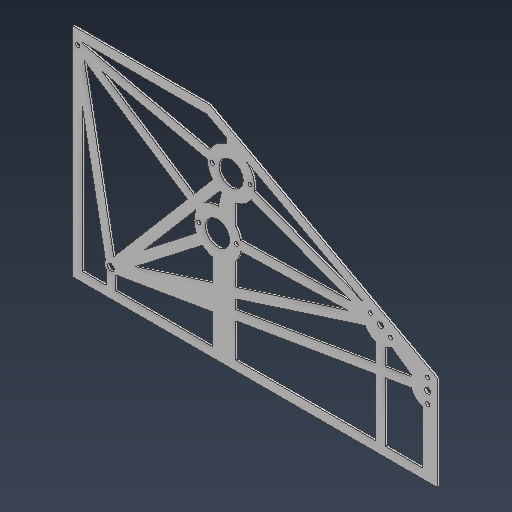
# Autodesk Inventor part: стенка
Saved by Autodesk Inventor 2025 (Build 290162000, 162)
## iProperties
Created: 2025-10-03
Part Number: стенка
Material: Типовые
Document SubType Name: Modeling
Designer: Phantom
Density: 1 g/cm^3
Appearance: По умолчанию
Author: Phantom
Autodesk Inventor part; units mm, degrees
ref_plane "YZ Plane" through (0, 0, 0) normal (1, 0, 0) x (0, 1, 0)
ref_plane "XZ Plane" through (0, 0, 0) normal (0, 1, 0) x (-1, 0, 0)
ref_plane "XY Plane" through (0, 0, 0) normal (0, 0, 1) x (1, 0, 0)
sketch "Эскиз1" plane through (0, 0, 0) normal (0, 0, 1) x (1, 0, 0)
  line L0 (0, 0) -> (380, 0)
  line L1 (380, 0) -> (380, 227)
  line L2 (380, 227) -> (0, 227)
  line L3 (0, 227) -> (0, 0)
  dimension "d0" = 380
  dimension "d1" = 227
  constraints: 8 end point, 2 parallel, 1 horizontal, 1 perpendicular
  measures "d0" distance of L2.end L1.end
  measures "d1" distance of L1.end L0.end
extrude "Выдавливание1" add sketch "Эскиз1" along normal blind 2
sketch "Эскиз2" plane through (0, 0, 2) normal (0, 0, 1) x (1, 0, 0)
  arc A0 (28.7106, 220.3235) -> (184.1593, 0) centre (184.1593, 165) ccw projected
  line L0 (380, 0) -> (380, 227) projected
  line L1 (380, 227) -> (0, 227) projected
  line L2 (0, 227) -> (0, 0) projected
  line L3 (0, 0) -> (380, 0) projected
  line L4 (19.1593, 227.9564) -> (19.1593, -26.9054)
  line L5 (0, 227) -> (0, 0) projected
  circle A1 centre (184.1593, 165) radius 165
  point P0 (19.1593, 165)
  point P1 (24, 227)
  point P2 (19.1593, 0)
  point P3 (19.1593, 227)
  point P4 (184.1593, 0)
  point P5 (28.7106, 220.3235)
  point P6 (31.2508, 227)
  constraints: 2 end point, 1 centre point, 1 coincident, 1 concentric, 1 parallel, 1 tangent
extrude "Выдавливание2" cut sketch "Эскиз2" against normal blind 10 contours L4 L3 L2 L1
sketch "Эскиз3" plane through (0, 0, 0) normal (0, 0, -1) x (-1, 0, 0)
  line L0 (-232.105, -3.3128) -> (-396.3335, -92) projected
  line L1 (-142.3437, 227) -> (-503.0133, 32.2299)
  line L2 (-14.2955, 176.8048) -> (-380, 176.8048) projected
  line L3 (-14.2955, 180) -> (-380, 180) projected
  line L4 (-380, 0) -> (-380, 176.8048) projected
  line L5 (-14.1593, 0) -> (-380, 0) projected
  line L6 (-14.1593, 0) -> (-14.1593, 170) projected
  arc A0 (-14.1593, 170) -> (-14.2955, 176.8048) centre (-184.1593, 170) ccw projected
  line L7 (-19.1593, 0) -> (-19.1593, 227) projected
  line L8 (-380, 227) -> (-19.1593, 227) projected
  line L9 (-380, 0) -> (-380, 227) projected
  line L10 (-19.1593, 0) -> (-380, 0) projected
  point P0 (0, 0)
  point P1 (-380, 98.66)
  dimension "d6" = 160
  constraints: 2 end point, 1 horizontal alignment, 1 parallel, 1 point on line, 1 other
  measures "d6" distance between parallel lines of L0 L1
extrude "Выдавливание3" cut sketch "Эскиз3" against normal blind 10 contours L1 L3 L9 L8 | L1 L2 L9 L3 | L1 L4 L2
sketch "Эскиз4" plane through (0, 0, 0) normal (0, 0, -1) x (-1, 0, 0)
  circle A0 centre (-150.9975, 115.172) radius 3 projected
  circle A1 centre (-150.9975, 115.172) radius 3.1
  circle A2 centre (-192.6104, 161.8048) radius 3.1 projected
  circle A3 centre (-192.6104, 161.8048) radius 3.1
  arc A4 (-37.1443, 30.0275) -> (-37.7482, 26.6179) centre (-39.8587, 28.75) ccw projected
  circle A5 centre (-39.8587, 28.75) radius 3.5
  point P0 (0, 0)
  dimension "d9" = 6.2
  dimension "d10" = 6.2
  dimension "d11" = 7
  constraints: 3 centre point, 3 coincident
  measures "d9" diameter of A1
  measures "d10" diameter of A3
  measures "d11" diameter of A5
extrude "Выдавливание5" cut sketch "Эскиз4" against normal blind 10 contours A0 | A2 | A5
sketch "Эскиз5" plane through (0, 0, 0) normal (0, 0, -1) x (-1, 0, 0)
  circle A0 centre (-184.1593, 165) radius 3.1
  circle A1 centre (-185.6251, 167.2025) radius 3.5
  circle A2 centre (-150.9975, 115.172) radius 3 projected
  circle A3 centre (-150.9975, 115.172) radius 62.5
  circle A4 centre (-182.6583, 169.0593) radius 3.5
  line L0 (-182.6583, 169.0593) -> (-162.6583, 169.0593)
  line L1 (-182.6583, 169.0593) -> (-162.6583, 169.0593) construction
  line L2 (-162.6583, 169.0593) -> (-162.6583, 176.0593)
  line L3 (-162.6583, 176.0593) -> (-181, 176.0593)
  circle A5 centre (-165.1036, 176.0593) radius 3.5
  point P0 (0, 0)
  point P1 (-187.1037, 164.0302)
  point P2 (-182.1279, 167.3417)
  point P3 (-185.8413, 167.604)
  point P4 (-185.7497, 170.7003)
  dimension "d20" = 7
  dimension "d21" = 20
  dimension "d22" = 0
  dimension "d23" = 7
  dimension "d24" = 7
  constraints: 8 end point, 4 centre point, 3 point on circle, 2 horizontal, 2 perpendicular, 1 coincident, 1 collinear, 1 point on line, 6 other
  measures "d20" diameter of A4
  measures "d21" distance of L0.start L0.end
  measures "d22" distance between parallel lines of L0 L1
  measures "d23" distance of L0.end L2.end
  measures "d24" diameter of A5
extrude "Выдавливание6" cut sketch "Эскиз5" against normal blind 7 contours A4 A1 A0 | A0 A1 L0 A4 | A1 A3 A0 | A1 A4 A3 A0 | A0 A3 A1 | L0 A3 A4 | A3 A1 A4 A0 | A3 A4 A0 | A0 A4 A1 A3 | A1 A4 A3 | A5 L3 A3 | A3 L3 L2 A5 | L2 L3 A3 A5 | A3 L3 A5 picked at (-181.7788, 166.0755) picked at (-184.2655, 167.3284) picked at (-187.1066, 167.9908) picked at (-185.4271, 167.6129) picked at (-185.0911, 169.2148)
sketch "Эскиз6" plane through (0, 0, 0) normal (0, 0, -1) x (-1, 0, 0)
  circle A0 centre (-369.8544, 82.5008) radius 25
  circle A1 centre (-320.7436, 116.97) radius 25
  circle A2 centre (-369.8544, 82.5008) radius 3.1
  circle A3 centre (-320.7436, 116.97) radius 3.1
  point P0 (0, 0)
  dimension "d25" = 6.2
  dimension "d26" = 6.2
  constraints: 4 centre point, 2 coincident, 4 other
  measures "d25" diameter of A2
  measures "d26" diameter of A3
extrude "Выдавливание7" cut sketch "Эскиз6" against normal blind 7 contours A2 | A3
sketch "Эскиз7" plane through (0, 0, 0) normal (0, 0, -1) x (-1, 0, 0)
  arc A0 (-185.8413, 167.604) -> (-185.7497, 170.7003) centre (-182.6583, 169.0593) ccw projected
  circle A1 centre (-192.6104, 161.8048) radius 3.1 projected
  arc A2 (-185.7497, 170.7003) -> (-187.1037, 164.0302) centre (-185.6251, 167.2025) ccw projected
  arc A3 (-185.8413, 167.604) -> (-187.1037, 164.0302) centre (-184.1593, 165) ccw projected
  point P0 (0, 0)
  point P1 (-181.1878, 165.8832)
  constraints: 1 other
extrude "Выдавливание8" add sketch "Эскиз7" against normal up to surface (2 mm away)
sketch "Эскиз8" plane through (19.1593, 0, 0) normal (0, -1, 0) x (1, 0, 0)
  line L0 (0, 2) -> (0, 0) projected
  line L1 (0, 0) -> (360.8407, 0) projected
  line L2 (360.8407, 0) -> (360.8407, 2) projected
  line L3 (0, 2) -> (360.8407, 2) projected
  point P0 (-19.1593, 0)
extrude "Выдавливание9" cut sketch "Эскиз8" against normal blind 0.313
sketch "Эскиз9" plane through (0, 0, 0) normal (0, 0, -1) x (-1, 0, 0)
  circle A0 centre (-165.1036, 176.0593) radius 3.5 projected
  circle A1 centre (-165.1036, 176.0593) radius 12.6
  circle A2 centre (-150.9975, 115.172) radius 3 projected
  circle A3 centre (-150.9975, 115.172) radius 12.6
  line L0 (-320.7437, 116.97) -> (-310.185, 122.672)
  line L1 (-142.3437, 227) -> (-380, 98.66) projected
  line L2 (-320.7437, 116.97) -> (-331.3025, 111.268)
  line L3 (-380, 0.313) -> (-19.1593, 0.313) projected
  line L4 (-19.1593, 0.313) -> (-19.1593, 227) projected
  line L5 (-142.3437, 227) -> (-19.1593, 227) projected
  line L6 (-142.3437, 227) -> (-380, 98.66) projected
  line L7 (-380, 0.313) -> (-380, 98.66) projected
  circle A4 centre (-150.9975, 115.172) radius 3 projected
  circle A5 centre (-39.8587, 28.75) radius 3.5 projected
  circle A6 centre (-165.1036, 176.0593) radius 3.5 projected
  circle A7 centre (-369.8544, 82.5008) radius 3.1 projected
  circle A8 centre (-320.7436, 116.97) radius 3.1 projected
  circle A9 centre (-331.3025, 111.268) radius 2.1
  circle A10 centre (-310.185, 122.672) radius 2.1
  line L8 (-369.8544, 82.5008) -> (-369.8544, 94.5008)
  line L9 (-369.8544, 94.5008) -> (-369.8544, 70.5008)
  circle A11 centre (-369.8544, 94.5008) radius 2.1
  circle A12 centre (-369.8544, 70.5008) radius 2.1
  circle A13 centre (-150.9975, 115.172) radius 3 projected
  line L10 (-150.9975, 115.172) -> (-170.5975, 115.172)
  circle A14 centre (-170.5975, 115.172) radius 2.1
  line L11 (-150.9975, 115.172) -> (-150.9975, 109.168)
  circle A15 centre (-131.3975, 115.172) radius 2.1
  circle A16 centre (-184.7036, 176.0593) radius 2.1
  circle A17 centre (-145.5036, 176.0593) radius 2.1
  point P0 (0, 0)
  dimension "d33" = 25.2
  dimension "d34" = 25.2
  dimension "d35" = 12
  dimension "d36" = 12
  dimension "d37" = 4.2
  dimension "d38" = 4.2
  dimension "d39" = 12
  dimension "d40" = 24
  dimension "d41" = 4.2
  dimension "d42" = 4.2
  dimension "d95" = 19.6
  dimension "d96" = 4.2
  dimension "d97" = 4.2
  constraints: 12 end point, 10 centre point, 7 coincident, 2 vertical, 1 collinear, 1 horizontal, 1 parallel, 1 point on line, 1 symmetric about line, 2 other
  measures "d33" diameter of A1
  measures "d34" diameter of A3
  measures "d35" distance of L0.start L0.end
  measures "d36" distance of L0.start L2.end
  measures "d37" diameter of A9
  measures "d38" diameter of A10
  measures "d39" distance of L8.start L8.end
  measures "d40" distance of L8.end L9.end
  measures "d41" diameter of A11
  measures "d42" diameter of A12
  measures "d95" distance of L10.start L10.end
  measures "d96" diameter of A14
  measures "d97" diameter of A16
extrude "Выдавливание10" cut sketch "Эскиз9" against normal through all contours A1 | A3 | A9 | A10 | A11 | A12 | A14 | A15 | A16 | A17
sketch "Эскиз10" plane through (0, 0, 0) normal (0, 0, -1) x (-1, 0, 0)
  line L0 (-0.0002, 0.3131) -> (-0.0002, 139.7466)
  arc A0 (-19.1593, 165) -> (-31.2508, 227) centre (-184.1593, 165) ccw projected
  line L1 (-19.1593, 0.313) -> (-19.1593, 227) projected
  line L2 (-0.0003, 0.313) -> (-0.0003, 165)
  arc A1 (-0.0003, 165) -> (-13.4958, 234.1991) centre (-184.1593, 165) ccw
  line L3 (-142.3437, 227) -> (-19.1593, 227) projected
  line L4 (-31.2508, 227) -> (23.6327, 227)
  line L5 (-19.1593, 0.313) -> (-0.0003, 0.313)
  line L6 (-0.0002, 0.3131) -> (-0.0002, 227.0001)
  line L7 (-0.0002, 227.0001) -> (-0.0003, 0.313)
  line L8 (-0.0003, 0.313) -> (-19.1593, 0.313)
  point P0 (0, 0)
  point P1 (-10.7507, 227)
  point P2 (-0.0002, 227)
  dimension "d45" = 19.159
  constraints: 14 end point, 2 horizontal, 2 point on circle, 2 vertical, 1 centre point, 4 other
  measures "d45" distance between parallel lines of L1 L2
extrude "Выдавливание11" add sketch "Эскиз10" against normal up to surface (2 mm away)
sketch "Эскиз11" plane through (0, 0, 0) normal (0, 0, -1) x (-1, 0, 0)
  circle A0 centre (-310.185, 122.672) radius 2.1 projected
  circle A1 centre (-369.8544, 70.5008) radius 2.1 projected
  circle A2 centre (-165.1036, 176.0593) radius 12.6 projected
  circle A3 centre (-331.3025, 111.268) radius 2.1 projected
  circle A4 centre (-369.8544, 94.5008) radius 2.1 projected
  circle A5 centre (-150.9975, 115.172) radius 12.6 projected
  line L0 (-380, 0.313) -> (-0.0003, 0.313) projected
  line L1 (-0.0002, 227) -> (-142.3437, 227) projected
  line L2 (-142.3437, 227) -> (-380, 98.66) projected
  line L3 (-380, 0.313) -> (-380, 98.66) projected
  circle A6 centre (-39.8587, 28.75) radius 3.5 projected
  circle A7 centre (-369.8544, 82.5008) radius 3.1 projected
  circle A8 centre (-320.7436, 116.97) radius 3.1 projected
  line L4 (-5.0003, 10.313) -> (-370, 10.313)
  line L5 (-139.8161, 217) -> (-5.0003, 217)
  line L6 (-150.9975, 115.172) -> (-150.9975, 10.313)
  line L7 (-165.1036, 176.0593) -> (-165.1036, 10.313)
  arc A9 (-333.9909, 112.141) -> (-309.4403, 125.3989) centre (-320.7436, 116.97) ccw
  arc A10 (-370, 68.4016) -> (-375, 95.6284) centre (-369.8544, 82.5008) ccw
  line L8 (-39.8587, 28.75) -> (-39.8587, 10.313)
  line L9 (-170.1036, 176.0593) -> (-170.1036, 5.313)
  line L10 (-160.1036, 176.0593) -> (-160.1036, 5.313)
  line L11 (-155.9975, 115.172) -> (-155.9975, 5.313)
  line L12 (-145.9975, 115.172) -> (-145.9975, 5.313)
  line L13 (-325.7436, 103.7863) -> (-325.7436, 10.313)
  line L14 (-34.8587, 28.75) -> (-34.8587, 5.313)
  line L15 (-44.8587, 28.75) -> (-44.8587, 5.313)
  line L16 (-320.7436, 102.87) -> (-320.7436, 10.313)
  line L17 (-369.8544, 68.4008) -> (-369.8544, 10.313)
  line L18 (-165.1036, 176.0593) -> (-150.9975, 115.172)
  line L19 (-150.9975, 115.172) -> (-39.8587, 28.75)
  line L20 (-165.1036, 176.0593) -> (-39.8587, 28.75)
  line L21 (-0.0003, 0.313) -> (-0.0002, 227) projected
  arc A11 (-5.0003, 214.0977) -> (-5.0003, 209.9025) centre (-5.1002, 212.0001) ccw
  arc A12 (-5.0003, 214.0977) -> (-5.0003, 209.9025) centre (-5.1002, 212.0001) ccw
  line L22 (-5.0003, 217) -> (-5.0003, 214.0977)
  line L23 (-372.6242, 91.2781) -> (-333.9909, 112.141)
  line L24 (-309.4403, 125.3989) -> (-139.8161, 217)
  line L25 (-370, 10.313) -> (-370, 68.4016)
  line L26 (-375, 95.6284) -> (-372.6242, 91.2781)
  line L27 (-5.1002, 212.0001) -> (-165.1036, 176.0593)
  line L28 (-5.1002, 212.0001) -> (-150.9975, 115.172)
  line L29 (-5.1002, 212.0001) -> (-39.8587, 28.75)
  line L30 (-355.757, 82.2299) -> (-39.8587, 28.75)
  line L31 (-364.8544, 69.3171) -> (-364.8544, 5.313)
  line L32 (-371.5779, 84.9564) -> (-370.9386, 85.4051)
  line L33 (-372.8544, 82.5008) -> (-372.8544, 81.7198)
  line L34 (-374.8544, 69.3171) -> (-374.8544, 5.313)
  line L35 (-356.6526, 87.4527) -> (-38.9995, 33.6757)
  line L36 (-356.7388, 77.325) -> (-40.6687, 23.816)
  line L37 (-165.1036, 176.0593) -> (-310.913, 120.7022)
  line L38 (-317.8454, 118.0703) -> (-320.7436, 116.97)
  line L39 (-150.9975, 115.172) -> (-306.7655, 118.8201)
  line L40 (-317.6437, 116.9372) -> (-320.7436, 116.97)
  line L41 (-320.7436, 116.97) -> (-317.7436, 116.0278)
  line L42 (-306.8284, 114.6946) -> (-39.8587, 28.75)
  line L43 (-317.7436, 116.97) -> (-317.7436, 116.0278)
  line L44 (-315.7436, 103.7863) -> (-315.7436, 5.313)
  line L45 (-356.1909, 85.9821) -> (-328.6622, 105.3036)
  line L46 (-319.6594, 114.0658) -> (-319.0201, 114.5145)
  line L47 (-358.3134, 90.6011) -> (-329.2168, 111.0229)
  line L48 (-323.2809, 115.1891) -> (-320.7436, 116.97)
  line L49 (-323.1063, 118.9769) -> (-322.467, 119.4255)
  line L50 (-308.4984, 109.9796) -> (-41.3638, 23.9818)
  line L51 (-306.9715, 119.9934) -> (-38.2994, 33.5007)
  line L52 (-151.0633, 110.1722) -> (-306.9989, 113.8242)
  line L53 (-150.8291, 120.1694) -> (-308.442, 123.8608)
  line L54 (-163.3289, 171.3849) -> (-309.1383, 116.0278)
  line L55 (-166.8783, 180.7338) -> (-312.6877, 125.3767)
  line L56 (-6.196, 216.8785) -> (-166.1994, 180.9378)
  line L57 (-4.0043, 207.1216) -> (-164.0078, 171.1809)
  line L58 (-7.865, 216.1661) -> (-153.7624, 119.338)
  line L59 (-161.2943, 179.2981) -> (-36.0494, 31.9887)
  line L60 (-154.0668, 111.2249) -> (-42.928, 24.8029)
  line L61 (-147.9282, 119.1191) -> (-36.7895, 32.6971)
  line L62 (-168.9129, 172.8206) -> (-43.668, 25.5113)
  line L63 (-2.3353, 207.8341) -> (-148.2326, 111.006)
  line L64 (-10.0126, 212.9319) -> (-44.7711, 29.6818)
  line L65 (-0.1878, 211.0683) -> (-34.9463, 27.8182)
  line L66 (-165.1036, 176.0593) -> (-165.1036, 237)
  line L67 (-170.1036, 176.0593) -> (-170.1036, 237)
  line L68 (-160.1036, 176.0593) -> (-160.1036, 237)
  circle A13 centre (-165.1036, 176.0593) radius 16.6
  circle A14 centre (-150.9975, 115.172) radius 16.6
  circle A15 centre (-39.8587, 28.75) radius 7
  circle A16 centre (-369.8544, 82.5008) radius 3.1 projected
  circle A17 centre (-369.8544, 82.5008) radius 18.1
  circle A18 centre (-320.7436, 116.97) radius 18.1
  circle A19 centre (-5.1002, 212.0001) radius 6.1
  line L69 (-160.2326, 177.1878) -> (-146.1265, 116.3005)
  line L70 (-169.9746, 174.9308) -> (-155.8685, 114.0435)
  circle A20 centre (-5.1002, 212.0001) radius 2.1
  circle A21 centre (-184.7036, 176.0593) radius 2.1 projected
  circle A22 centre (-145.5036, 176.0593) radius 2.1 projected
  circle A23 centre (-131.3975, 115.172) radius 2.1 projected
  circle A24 centre (-170.5975, 115.172) radius 2.1 projected
  circle A25 centre (-165.1036, 176.0593) radius 24.65
  circle A26 centre (-150.9975, 115.172) radius 24.65
  line L71 (-361.1858, 94.6937) -> (-332.0893, 115.1155)
  line L72 (-10.0002, 251) -> (-10.0003, -70)
  point P0 (0, 0)
  point P1 (-34.0334, 32.6314)
  point P2 (-34.8587, 23.851)
  point P3 (-34.8587, 10.313)
  point P4 (-44.8587, 23.851)
  point P5 (-45.5236, 24.6379)
  point P6 (-145.9975, 41.6476)
  point P7 (-145.9975, 10.313)
  point P8 (-44.8587, 10.313)
  point P9 (-155.9975, 43.3405)
  point P10 (-160.1036, 44.0357)
  point P11 (-160.1036, 10.313)
  point P12 (-155.9975, 10.313)
  point P13 (-155.9975, 60.8855)
  point P14 (-160.1036, 62.2073)
  point P15 (-160.1036, 54.178)
  point P16 (-155.9975, 53.4828)
  point P17 (-155.9975, 99.3429)
  point P18 (-160.1036, 101.2926)
  point P19 (-160.1036, 72.7127)
  point P20 (-155.9975, 71.3909)
  point P21 (-141.571, 101.5081)
  point P22 (-145.9975, 99.3429)
  point P23 (-145.9975, 68.1716)
  point P24 (-65.2856, 42.1883)
  point P25 (-135.4324, 109.4023)
  point P26 (-75.1173, 62.501)
  point P27 (-127.8553, 124.5299)
  point P28 (-135.0438, 119.759)
  point P29 (-159.4411, 129.4642)
  point P30 (-160.1036, 132.3239)
  point P31 (-160.1036, 129.0514)
  point P32 (-156.66, 161.7672)
  point P33 (-149.6991, 131.7211)
  point P34 (-140.5736, 128.091)
  point P35 (-134.3786, 132.2024)
  point P36 (-158.6597, 160.7611)
  point P37 (-39.2227, 35.721)
  point P38 (-43.8582, 34.4949)
  point P39 (-12.2244, 201.271)
  point P40 (-119.4643, 130.0988)
  point P41 (-148.5635, 174.6501)
  point P42 (-151.0411, 167.2385)
  point P43 (-125.9876, 137.7713)
  point P44 (-30.4403, 201.1835)
  point P45 (-160.1036, 206.0443)
  point P46 (-160.1036, 191.8884)
  point P47 (-150.7552, 184.4069)
  point P48 (-9.6053, 216.1127)
  point P49 (-5.0003, 218.0993)
  point P50 (-305.8915, 127.3154)
  point P51 (-306.2552, 127.8188)
  point P52 (-181.6767, 175.1155)
  point P53 (-170.1036, 191.8884)
  point P54 (-170.1036, 200.644)
  point P55 (-302.7058, 118.4699)
  point P56 (-303.9638, 123.7559)
  point P57 (-170.1036, 120.6208)
  point P58 (-170.1036, 160.2302)
  point P59 (-178.1274, 165.7666)
  point P60 (-170.1036, 110.6181)
  point P61 (-286.3025, 113.3395)
  point P62 (-170.1036, 75.932)
  point P63 (-304.6264, 108.7331)
  point P64 (-315.7436, 99.5743)
  point P65 (-315.7436, 80.527)
  point P66 (-170.1036, 55.8709)
  point P67 (-170.1036, 65.4266)
  point P68 (-337.5397, 110.2246)
  point P69 (-360.3516, 97.9056)
  point P70 (-325.7436, 99.5743)
  point P71 (-332.1097, 102.8838)
  point P72 (-352.7434, 88.4018)
  point P73 (-352.25, 86.7074)
  point P74 (-325.7436, 82.2199)
  point P75 (-352.7275, 76.6459)
  point P76 (-364.8544, 65.1052)
  point P77 (-364.8544, 10.313)
  point P78 (-325.7436, 72.0777)
  point P79 (-315.7436, 70.3847)
  point P80 (-315.7436, 10.313)
  point P81 (-170.1036, 10.313)
  point P82 (-170.1036, 45.7286)
  point P83 (-107.4976, 45.2721)
  point P84 (-145.9975, 57.6662)
  point P85 (-145.9975, 51.7899)
  point P86 (-5.0003, 214.0977)
  point P87 (-5.0003, 209.9025)
  point P88 (-160.1036, 138.0784)
  point P89 (-161.3163, 137.5583)
  point P90 (-151.5743, 139.8153)
  point P91 (-133.6509, 132.6854)
  point P92 (-153.2779, 154.4312)
  point P93 (-154.7848, 153.6731)
  point P94 (-155.9975, 91.0344)
  point P95 (-160.1036, 92.2656)
  point P96 (-135.0121, 96.4079)
  point P97 (-145.9975, 91.0344)
  point P98 (-128.8736, 104.3021)
  point P99 (-128.1212, 124.3534)
  point P100 (-140.457, 176.471)
  point P101 (-145.6593, 160.9087)
  point P102 (-160.1036, 200.1969)
  point P103 (-142.6487, 186.2279)
  point P104 (-189.4443, 172.1665)
  point P105 (-170.1036, 200.1969)
  point P106 (-175.0114, 120.7358)
  point P107 (-170.1036, 130.7469)
  point P108 (-170.1036, 151.9218)
  point P109 (-185.8949, 162.8176)
  point P110 (-170.1036, 99.5971)
  point P111 (-175.2455, 110.7385)
  point P112 (-42.8225, 39.955)
  point P113 (-370, 64.4014)
  point P114 (-137.3539, 135.7019)
  point P115 (-147.754, 123.3256)
  point P116 (-128.5403, 125.3356)
  point P117 (-155.5907, 157.1514)
  point P118 (-170.1036, 168.8128)
  point P119 (-289.6647, 123.421)
  point P120 (-358.4882, 96.587)
  point P121 (-337.8546, 111.069)
  point P122 (-171.5927, 199.8399)
  point P123 (-181.4298, 194.5276)
  point P124 (-170.1036, 179.5093)
  point P125 (-301.8914, 129.4755)
  point P126 (-364.6278, 95.5964)
  point P127 (-160.1036, 182.307)
  point P128 (-8.5946, 217)
  point P129 (-34.8587, 28.28)
  point P130 (-344.1229, 106.6695)
  point P131 (-10.0003, 10.313)
  point P132 (-10.0002, 159.3362)
  point P133 (-10.0002, 216.024)
  point P134 (-10.0002, 217)
  dimension "d49" = 28.2
  dimension "d50" = 28.2
  dimension "d51" = 5
  dimension "d52" = 5
  dimension "d53" = 5
  dimension "d54" = 5
  dimension "d59" = 5
  dimension "d60" = 5
  dimension "d63" = 5
  dimension "d64" = 5
  dimension "d65" = 5
  dimension "d66" = 5
  dimension "d67" = 5
  dimension "d68" = 5
  dimension "d69" = 5
  dimension "d70" = 5
  dimension "d71" = 5
  dimension "d72" = 5
  dimension "d73" = 5
  dimension "d74" = 5
  dimension "d75" = 5
  dimension "d76" = 5
  dimension "d77" = 5
  dimension "d78" = 5
  dimension "d79" = 5
  dimension "d80" = 5
  dimension "d81" = 5
  dimension "d82" = 5
  dimension "d83" = 33.2
  dimension "d84" = 33.2
  dimension "d85" = 14
  dimension "d87" = 36.2
  dimension "d88" = 36.2
  dimension "d89" = 12.2
  dimension "d90" = 5
  dimension "d91" = 5
  dimension "d98" = 49.3
  dimension "d99" = 49.3
  dimension "d100" = 5
  dimension "d101" = 5
  dimension "d102" = 5
  dimension "d103" = 5
  dimension "d104" = 5
  dimension "d106" = 0
  dimension "d108" = 5
  dimension "d109" = 10
  dimension "d110" = 10
  dimension "d111" = 10
  dimension "d112" = 10
  dimension "d113" = 10
  dimension "d114" = 10
  constraints: 136 end point, 44 parallel, 11 centre point, 11 coincident, 11 point on circle, 6 point on line, 6 vertical, 1 concentric, 1 perpendicular, 35 other
  measures "d51" distance between parallel lines of L7 L9
  measures "d52" distance between parallel lines of L7 L10
  measures "d53" distance between parallel lines of L6 L11
  measures "d54" distance between parallel lines of L6 L12
  measures "d59" distance between parallel lines of L8 L14
  measures "d60" distance between parallel lines of L8 L15
  measures "d63" distance between parallel lines of L30 L35
  measures "d64" distance between parallel lines of L30 L36
  measures "d65" distance between parallel lines of L42 L50
  measures "d66" distance between parallel lines of L42 L51
  measures "d67" distance between parallel lines of L39 L52
  measures "d68" distance between parallel lines of L39 L53
  measures "d69" distance between parallel lines of L37 L54
  measures "d70" distance between parallel lines of L37 L55
  measures "d71" distance between parallel lines of L27 L56
  measures "d72" distance between parallel lines of L27 L57
  measures "d73" distance between parallel lines of L28 L58
  measures "d74" distance between parallel lines of L20 L59
  measures "d75" distance between parallel lines of L19 L60
  measures "d76" distance between parallel lines of L19 L61
  measures "d77" distance between parallel lines of L20 L62
  measures "d78" distance between parallel lines of L28 L63
  measures "d79" distance between parallel lines of L29 L64
  measures "d80" distance between parallel lines of L29 L65
  measures "d81" distance between parallel lines of L66 L67
  measures "d82" distance between parallel lines of L66 L68
  measures "d83" diameter of A13
  measures "d84" diameter of A14
  measures "d85" diameter of A15
  measures "d87" diameter of A17
  measures "d88" diameter of A18
  measures "d89" diameter of A19
  measures "d90" distance between parallel lines of L18 L69
  measures "d91" distance between parallel lines of L18 L70
  measures "d98" diameter of A25
  measures "d99" diameter of A26
  measures "d100" distance between parallel lines of L13 L16
  measures "d101" distance between parallel lines of L16 L44
  measures "d102" distance between parallel lines of L17 L31
  measures "d103" distance between parallel lines of L34 L17
  measures "d104" distance between parallel lines of L47 L45
  measures "d106" distance from line of A7.centre L17
  measures "d108" distance between parallel lines of L47 L71
  measures "d109" distance between parallel lines of L0 L4
  measures "d110" distance between parallel lines of L3 L25
  measures "d111" distance between parallel lines of L2 L23
  measures "d112" distance between parallel lines of L2 L24
  measures "d113" distance between parallel lines of L1 L5
  measures "d114" distance between parallel lines of L21 L72
extrude "Выдавливание12" cut sketch "Эскиз11" against normal blind 36.2 contours L54 A25 L9 A26 L53 | L24 A25 L55 | L52 A26 L9 L51 | L50 L9 L35 L44 A18 | L24 L5 L72 L56 A25 L68 | A18 L13 L35 A17 L45 | A25 L62 A26 L69 | L36 L9 L4 L44 | L12 A26 L60 L51 | L57 L58 L59 A25 | L4 L14 A15 L65 L72 | A17 L36 L13 L4 L31 | A20 A11 L29 L27 | A26 L63 L62 L61 | L27 L28 A11 | L4 L12 L36 A15 L15 | L28 L29 A11 | L63 L64 L59
equation "\"d16\" = d24"
equation "\"d27\" = d24"
